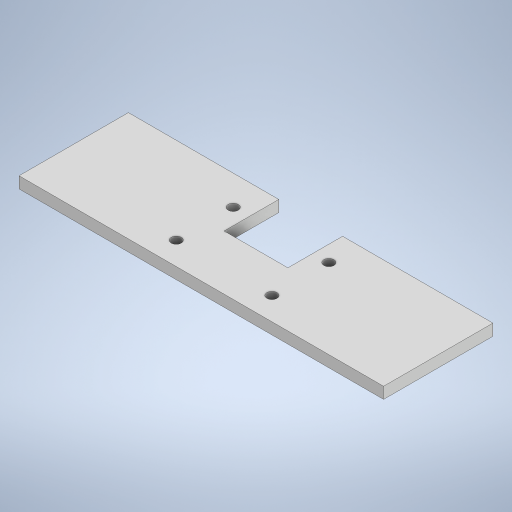
# Autodesk Inventor part: kamera2
Saved by Autodesk Inventor 2024.1 (Build 281209000, 209)
## iProperties
Created: 2025-01-07
Part Number: kamera2
Material: Všeobecné
Document SubType Name: Modeling
Designer: elias
Density: 1 g/cm^3
Appearance: Výchozí
Author: elias
Autodesk Inventor part; units mm, degrees
ref_plane "YZ Plane" through (0, 0, 0) normal (1, 0, 0) x (0, 1, 0)
ref_plane "XZ Plane" through (0, 0, 0) normal (0, 1, 0) x (-1, 0, 0)
ref_plane "XY Plane" through (0, 0, 0) normal (0, 0, 1) x (1, 0, 0)
sketch "Náčrt1" plane through (0, 0, 0) normal (0, 0, 1) x (1, 0, 0)
  line L0 (0, 0) -> (0, 32)
  line L1 (0, 0) -> (40, 0)
  circle A0 centre (10.5, 5) radius 1.1
  circle A1 centre (10.5, 17.5) radius 1.1
  line L2 (0, 12) -> (7, 12)
  line L3 (7, 12) -> (7, 24)
  line L4 (7, 24) -> (40, 24)
  line L5 (40, 24) -> (40, 0)
  line L6 (0, 0) -> (-40, 0)
  circle A2 centre (-10.5, 5) radius 1.1
  circle A3 centre (-10.5, 17.5) radius 1.1
  line L7 (0, 12) -> (-7, 12)
  line L8 (-7, 12) -> (-7, 24)
  line L9 (-7, 24) -> (-40, 24)
  line L10 (-40, 24) -> (-40, 0)
  dimension "d0" = 32
  dimension "d1" = 40
  dimension "d2" = 2.2
  dimension "d3" = 5
  dimension "d4" = 10.5
  dimension "d5" = 2.2
  dimension "d6" = 12.5
  dimension "d7" = 12
  dimension "d8" = 7
  dimension "d9" = 12
  constraints: 22 end point, 6 symmetric about line, 4 centre point, 3 horizontal, 2 perpendicular, 1 point on line, 1 vertical, 2 other
  measures "d0" distance of L0.start L0.end
  measures "d1" distance of L0.start L1.end
  measures "d2" diameter of A0
  measures "d3" distance from line of L1 A0.centre
  measures "d4" distance from line of A0.centre L0
  measures "d5" diameter of A1
  measures "d6" distance of A0.centre A1.centre
  measures "d7" distance between parallel lines of L1 L2
  measures "d8" distance of L2.start L2.end
  measures "d9" distance of L2.end L3.end
extrude "Vysunutí1" add sketch "Náčrt1" along normal blind 2.5
